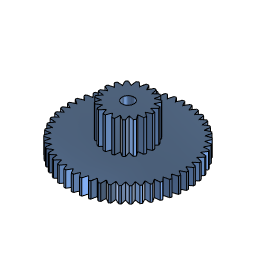
MG996R_Gear_3 v5 (Autodesk Fusion 360 design; units mm, degrees)
Autodesk Fusion 360 part; units mm, degrees
sketch "Sketch1" plane through (0, 0, 0) normal (0, 0, 1) x (1, 0, 0)
  circle A0 centre (0, 0) radius 3
  circle A1 centre (0, 0) radius 7.5
  dimension "d1" = 6
  dimension "d2" = 15
  constraint coincident A0.centre A1.centre
  constraint concentric A0 A1
  measures "d1" diameter of A0
  measures "d2" diameter of A1
extrude "Extrude1" add sketch "Sketch1" along normal blind 6 contours A0
extrude "Extrude2" add sketch "Sketch1" along normal blind 2
sketch "Sketch2" plane through (0, 0, 6) normal (0, 0, 1) x (-1, 0, 0)
  circle A0 centre (0, 0) radius 3
  circle A1 centre (0, 0) radius 0.75
  dimension "d7" = 1.5
  constraint coincident A0.centre A1.centre
  measures "d7" diameter of A1
extrude "Extrude3" cut sketch "Sketch2" against normal blind 14 contours A1
sketch "Sketch3" plane through (0, 0, 2) normal (0, 0, 1) x (-1, 0, 0)
  circle A0 centre (0, 0) radius 3
  circle A1 centre (0, 0) radius 7.5
  circle A2 centre (0, 0) radius 7.5
  line L0 (0.35, -7.4918) -> (0, -6.8856)
  line L1 (0, -6.8856) -> (-0.35, -7.4918)
  dimension "d10" = 0.7
  dimension "d11" = 0.7
  constraint concentric A0 A2
  constraint equal A1 A2
  constraint coincident A2 L0.start
  constraint coincident A2 L1.end
  constraint equal L0 L1
  constraint vertical A0.centre L0.end
  measures "d10" horizontal distance of L0.start L1.end
  measures "d11" distance of L0.start L0.end
extrude "Extrude4" cut sketch "Sketch3" against normal blind 5.5 contours A1 A2 L0 L1 picked at (0, -7.2946)
pattern_circular "C-Pattern1" count 50 over 360 about axis through (0, 0, 6) along (0, 0, -1) of "Extrude4"
sketch "Sketch4" plane through (0, 0, 6) normal (0, 0, 1) x (-1, 0, 0)
  circle A0 centre (0, 0) radius 0.75
  circle A1 centre (0, 0) radius 3
  circle A2 centre (0, 0) radius 3
  line L0 (0.35, -2.9795) -> (0, -2.3733)
  line L1 (0, -2.3733) -> (-0.35, -2.9795)
  dimension "d16" = 0.7
  dimension "d17" = 0.7
  constraint concentric A0 A2
  constraint equal A1 A2
  constraint coincident A1 L0.start
  constraint coincident A2 L1.end
  constraint vertical A0.centre L0.end
  constraint equal L0 L1
  measures "d16" distance of L0.start L0.end
  measures "d17" horizontal distance of L0.start L1.end
extrude "Extrude5" cut sketch "Sketch4" against normal blind 4 contours A1 A2 L0 L1 picked at (0, -2.7896)
pattern_circular "C-Pattern2" count 19 over 360 about axis through (0, 0, 6) along (0, 0, -1) of "Extrude5"
